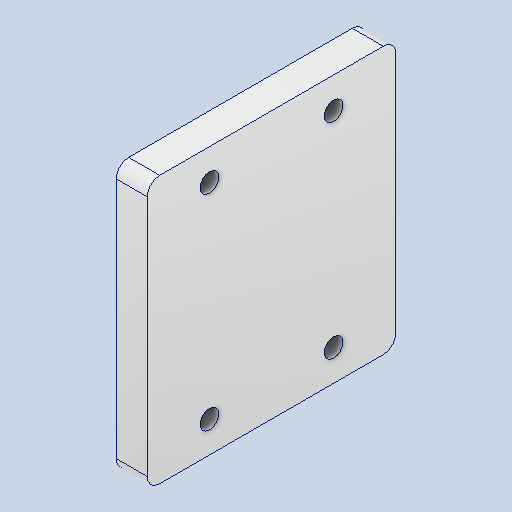
# Autodesk Inventor part: dribl-v4-Plate-3
Saved by Autodesk Inventor 2025.2 (Build 292293000, 293)
## iProperties
Created: 2025-05-14
Part Number: dribl-v4-Plate-3
Material: アルミニウム 6061
Document SubType Name: Modeling
Designer: haruy
Density: 2.7 g/cm^3
Appearance: アルミニウム - フラット
Author: haruy
Autodesk Inventor part; units mm, degrees
ref_plane "YZ Plane" through (0, 0, 0) normal (1, 0, 0) x (0, 1, 0)
ref_plane "XZ Plane" through (0, 0, 0) normal (0, 1, 0) x (-1, 0, 0)
ref_plane "XY Plane" through (0, 0, 0) normal (0, 0, 1) x (1, 0, 0)
sketch "スケッチ2" plane through (0, 0, 0) normal (1, 0, 0) x (0, 1, 0)
  line L0 (-303.8319, -112.1762) -> (-303.8319, -45.1762)
  line L1 (-303.8319, -98.1762) -> (-260.8319, -98.1762)
  line L2 (-260.8319, -98.1762) -> (-260.8319, -138.1762)
  line L3 (-260.8319, -138.1762) -> (-303.8319, -138.1762)
  line L4 (-303.8319, -138.1762) -> (-303.8319, -98.1762)
  line L5 (-260.8319, -97.1762) -> (-260.8319, -127.1762)
  line L6 (-303.8319, -97.1762) -> (-260.8319, -97.1762)
  line L7 (-303.8319, -127.1762) -> (-303.8319, -60.1762)
  line L8 (-303.8319, -118.1762) -> (-260.8319, -118.1762)
  circle A0 centre (-298.8319, -128.1762) radius 1.5
  line L9 (-282.3319, -138.1762) -> (-282.3319, -98.1762)
  circle A1 centre (-298.8319, -108.1762) radius 1.5
  circle A2 centre (-265.8319, -108.1762) radius 1.5
  circle A3 centre (-265.8319, -128.1762) radius 1.5
  line L10 (-303.8319, -127.1762) -> (-293.8319, -127.1762)
  line L11 (-293.8319, -127.1762) -> (-293.8319, -138.1762)
  line L12 (-293.8319, -138.1762) -> (-303.8319, -138.1762)
  line L13 (-303.8319, -138.1762) -> (-303.8319, -127.1762)
  line L14 (-270.8319, -127.1762) -> (-270.8319, -60.1762)
  line L15 (-260.8319, -138.1762) -> (-270.8319, -138.1762)
  line L16 (-270.8319, -138.1762) -> (-270.8319, -127.1762)
  line L17 (-270.8319, -127.1762) -> (-260.8319, -127.1762)
  line L18 (-260.8319, -127.1762) -> (-260.8319, -138.1762)
  line L19 (-169.3319, 147.8238) -> (184.6681, 147.8238)
  line L20 (7.6681, 147.8238) -> (7.6681, -98.1762)
  line L21 (319.1681, -98.1762) -> (276.1681, -98.1762)
  line L22 (319.1681, -138.1762) -> (319.1681, -98.1762)
  line L23 (276.1681, -138.1762) -> (319.1681, -138.1762)
  line L24 (309.1681, -127.1762) -> (309.1681, -138.1762)
  line L25 (319.1681, -127.1762) -> (309.1681, -127.1762)
  circle A4 centre (314.1681, -128.1762) radius 1.5
  circle A5 centre (314.1681, -108.1762) radius 1.5
  circle A6 centre (281.1681, -108.1762) radius 1.5
  circle A7 centre (281.1681, -128.1762) radius 1.5
  line L26 (286.1681, -127.1762) -> (276.1681, -127.1762)
  line L27 (286.1681, -138.1762) -> (286.1681, -127.1762)
  line L28 (276.1681, -98.1762) -> (276.1681, -138.1762)
  point P0 (0, 0)
  point P1 (-272.3319, -112.1762)
  point P2 (-270.8319, -138.1762)
  dimension "d11" = 40
  dimension "d12" = 0
  dimension "d13" = 1
  dimension "d14" = 20
  dimension "d15" = 3
  dimension "d16" = 5
  dimension "d17" = 10
  dimension "d18" = 10
  constraints: 58 end point, 17 symmetric about line, 8 centre point, 6 parallel, 5 point on line, 4 perpendicular, 3 horizontal, 3 midpoint, 1 vertical, 7 other
  measures "d11" distance of L1.end L2.end
  measures "d12" distance between parallel lines of L2 L5
  measures "d13" distance between parallel lines of L1 L6
  measures "d14" distance between parallel lines of L8 L1
  measures "d15" diameter of A0
  measures "d16" distance from line of L4 A0.centre
  measures "d17" distance from line of L8 A0.centre
  measures "d18" distance of L11.end L12.end
extrude "押し出し2" add sketch "スケッチ2" along normal blind 5 contours L22 L25 A4 L24 L23 L27 L26 A7 L28 L21 | L22 L23 L24 L25 A4 | L26 A7 L27 L23 L28
fillet "フィレット2" radius 2 4 edges at (2.5, 319.1681, -98.1762) (2.5, 319.1681, -138.1762) (2.5, 276.1681, -98.1762) (2.5, 276.1681, -138.1762)
